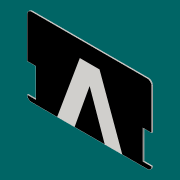
# Autodesk Inventor part: card-00
Saved by Autodesk Inventor 2016 (Build 200138000, 138)
## iProperties
Created: 2015-10-05
Part Number: card-00
Material: ABS Plastic
Document SubType Name: Modeling
Designer: Sawaiz
Density: 1.06 g/cm^3
Appearance: Smooth - White
Mass: 3.5118 g
Surface Area: 89.4505 cm^2
Volume: 3.31302 cm^3
Author: Sawaiz
Autodesk Inventor part; units mm, degrees
ref_plane "YZ Plane" through (0, 0, 0) normal (1, 0, 0) x (0, 1, 0)
ref_plane "XZ Plane" through (0, 0, 0) normal (0, 1, 0) x (-1, 0, 0)
ref_plane "XY Plane" through (0, 0, 0) normal (0, 0, 1) x (1, 0, 0)
sketch "Sketch1" plane through (0, 0, 0) normal (0, 1, 0) x (-1, 0, 0)
  line L0 (42.8, -26.99) -> (-42.8, -26.99)
  line L1 (-42.8, -26.99) -> (-42.8, 26.99)
  line L2 (-42.8, 26.99) -> (42.8, 26.99)
  line L3 (42.8, 26.99) -> (42.8, -26.99)
  line L4 (42.8, -26.99) -> (-42.8, 26.99) construction
  line L5 (-42.8, -26.99) -> (42.8, 26.99) construction
  point P0 (0, 0)
  dimension "d0" = 85.6
  dimension "d1" = 53.98
  constraints: 12 end point, 2 midpoint, 2 parallel, 1 horizontal, 1 perpendicular
  measures "d0" distance of L1.end L2.end
  measures "d1" distance of L0.end L1.end
extrude "Extrusion1" add sketch "Sketch1" along normal blind 0.76
fillet "Fillet1" radius 2.88 4 edges at (42.8, 0.38, 26.99) (42.8, 0.38, -26.99) (-42.8, 0.38, 26.99) (-42.8, 0.38, -26.99)
sketch "Sketch2" plane through (0, 0, 0) normal (0, -1, 0) x (1, 0, 0)
  arc A0 (-42.8, -24.11) -> (-39.92, -26.99) centre (-39.92, -24.11) ccw projected
  line L0 (-39.92, -26.99) -> (39.92, -26.99) projected
  arc A1 (39.92, -26.99) -> (42.8, -24.11) centre (39.92, -24.11) ccw projected
  line L1 (42.8, -24.11) -> (42.8, 24.11) projected
  arc A2 (42.8, 24.11) -> (39.92, 26.99) centre (39.92, 24.11) ccw projected
  line L2 (39.92, 26.99) -> (-39.92, 26.99) projected
  arc A3 (-39.92, 26.99) -> (-42.8, 24.11) centre (-39.92, 24.11) ccw projected
  line L3 (-42.8, 24.11) -> (-42.8, -24.11) projected
  line L4 (-42.8, 24.11) -> (-42.8, -24.11) projected
  line L5 (-42.8, -3.99) -> (-37.212, -3.99)
  line L6 (-37.212, -3.99) -> (-37.212, -23.99)
  line L7 (-37.212, -23.99) -> (-42.8, -23.99)
  line L8 (-42.8, -23.99) -> (-42.8, -3.99)
  line L9 (42.8, 24.11) -> (42.8, -24.11) projected
  line L10 (42.8, -23.99) -> (37.212, -23.99)
  line L11 (37.212, -23.99) -> (37.212, -3.99)
  line L12 (37.212, -3.99) -> (42.8, -3.99)
  line L13 (42.8, -3.99) -> (42.8, -23.99)
  point P0 (0, 0)
  dimension "d5" = 5.588
  dimension "d6" = 5.588
  dimension "d7" = 3
  dimension "d8" = 3
  dimension "d9" = 20
  dimension "d10" = 20
  constraints: 16 end point, 4 parallel, 2 horizontal, 2 perpendicular, 2 point on line
  measures "d5" distance between parallel lines of L6 L3
  measures "d6" distance of L11.end L12.end
  measures "d7" distance between parallel lines of L0 L7
  measures "d8" distance between parallel lines of L0 L10
  measures "d9" distance between parallel lines of L10 L12
  measures "d10" distance between parallel lines of L7 L5
extrude "Extrusion2" cut sketch "Sketch2" against normal through all contours L3 L5 L6 L7 | L10 L11 L12 L1
sketch "Sketch3" plane through (42.8, 0, 24.11) normal (1, 0, 0) x (0, 0, -1)
  line L0 (51.1, 0) -> (51.1, 0.76) projected
  line L1 (51.1, 0) -> (51.1, 0.76)
  line L2 (48.1, 0.76) -> (48.1, 0)
  line L3 (48.1, 0) -> (51.1, 0.76) construction
  line L4 (51.1, 0) -> (48.1, 0.76) construction
  line L5 (51.1, 0) -> (48.22, 0) projected
  arc A0 (48.1489, 0.76) -> (48.1489, 0) centre (49.6, 0.38) ccw
  arc A1 (51.0511, 0) -> (51.0511, 0.76) centre (49.6, 0.38) ccw
  line L6 (48.1, 0) -> (48.1489, 0)
  line L7 (51.0511, 0) -> (51.1, 0)
  line L8 (51.1, 0.76) -> (51.0511, 0.76)
  line L9 (48.1489, 0.76) -> (48.1, 0.76)
  point P0 (24.11, 0)
  point P1 (48.1, 0.38)
  point P2 (51.1, 0.38)
  dimension "d14" = 3
  dimension "d15" = 0.76
  dimension "d16" = 1.5
  dimension "d17" = 1.5
  dimension "d18" = 1.5
  constraints: 16 end point, 6 point on circle, 5 parallel, 4 midpoint, 3 collinear, 2 centre point, 2 horizontal, 2 perpendicular, 1 point on line
  measures "d14" distance of L2.start L1.end
  measures "d15" distance of L0.start L1.end
  measures "d16" radius of A0
  measures "d17" distance from line of L0 A0.centre
  measures "d18" radius of A1
extrude "Extrusion3" cut sketch "Sketch3" against normal up to surface (5.588 mm away)
mirror "Mirror1" about plane through (0, 0, 0) normal (1, 0, 0) of "Extrusion3"
sketch "Sketch4" plane through (0, 0, 0) normal (0, -1, 0) x (1, 0, 0)
  line L0 (-37.212, -24.0389) -> (-42.8, -24.0389) projected
  line L1 (-42.8, -24.0389) -> (-42.8, -24.11) projected
  arc A0 (-42.8, -24.11) -> (-40.4486, -26.9411) centre (-39.92, -24.11) ccw projected
  line L2 (-40.4486, -26.9411) -> (-37.212, -26.9411) projected
  line L3 (-37.212, -26.9411) -> (-37.212, -26.99) projected
  line L4 (-37.212, -26.99) -> (37.212, -26.99) projected
  line L5 (37.212, -26.99) -> (37.212, -26.9411) projected
  line L6 (37.212, -26.9411) -> (40.4486, -26.9411) projected
  arc A1 (40.4486, -26.9411) -> (42.8, -24.11) centre (39.92, -24.11) ccw projected
  line L7 (42.8, -24.11) -> (42.8, -24.0389) projected
  line L8 (42.8, -24.0389) -> (37.212, -24.0389) projected
  line L9 (37.212, -24.0389) -> (37.212, -3.99) projected
  line L10 (37.212, -3.99) -> (42.8, -3.99) projected
  line L11 (42.8, -3.99) -> (42.8, 24.11) projected
  arc A2 (42.8, 24.11) -> (39.92, 26.99) centre (39.92, 24.11) ccw projected
  line L12 (39.92, 26.99) -> (-39.92, 26.99) projected
  arc A3 (-39.92, 26.99) -> (-42.8, 24.11) centre (-39.92, 24.11) ccw projected
  line L13 (-42.8, 24.11) -> (-42.8, -3.99) projected
  line L14 (-42.8, -3.99) -> (-37.212, -3.99) projected
  line L15 (-37.212, -3.99) -> (-37.212, -24.0389) projected
  line L16 (39.92, 26.99) -> (-39.92, 26.99) projected
  line L17 (42.8, -3.99) -> (42.8, 24.11) projected
  line L18 (-42.8, 24.11) -> (-42.8, -3.99) projected
  line L19 (-42.8, 26.99) -> (42.8, 26.99) construction
  line L20 (42.8, 26.99) -> (42.8, -27.0263) construction
  line L21 (42.8, -27.0263) -> (-42.8, -27.0263) construction
  line L22 (-42.8, -27.0263) -> (-42.8, 26.99) construction
  point P0 (0, 0)
  constraints: 3 collinear, 2 other
decal "Decal1"
sketch "Sketch5" plane through (0, 0.76, 0) normal (0, 1, 0) x (1, 0, 0)
  line L0 (-42.8, 24.0389) -> (-37.212, 24.0389) projected
  line L1 (-37.212, 24.0389) -> (-37.212, 3.99) projected
  line L2 (-37.212, 3.99) -> (-42.8, 3.99) projected
  line L3 (-42.8, 3.99) -> (-42.8, -24.11) projected
  arc A0 (-42.8, -24.11) -> (-39.92, -26.99) centre (-39.92, -24.11) ccw projected
  line L4 (-39.92, -26.99) -> (39.92, -26.99) projected
  arc A1 (39.92, -26.99) -> (42.8, -24.11) centre (39.92, -24.11) ccw projected
  line L5 (42.8, -24.11) -> (42.8, 3.99) projected
  line L6 (42.8, 3.99) -> (37.212, 3.99) projected
  line L7 (37.212, 3.99) -> (37.212, 24.0389) projected
  line L8 (37.212, 24.0389) -> (42.8, 24.0389) projected
  line L9 (42.8, 24.0389) -> (42.8, 24.11) projected
  arc A2 (42.8, 24.11) -> (40.4486, 26.9411) centre (39.92, 24.11) ccw projected
  line L10 (40.4486, 26.9411) -> (37.212, 26.9411) projected
  line L11 (37.212, 26.9411) -> (37.212, 26.99) projected
  line L12 (37.212, 26.99) -> (-37.212, 26.99) projected
  line L13 (-37.212, 26.99) -> (-37.212, 26.9411) projected
  line L14 (-37.212, 26.9411) -> (-40.4486, 26.9411) projected
  arc A3 (-40.4486, 26.9411) -> (-42.8, 24.11) centre (-39.92, 24.11) ccw projected
  line L15 (-42.8, 24.11) -> (-42.8, 24.0389) projected
  line L16 (-42.8, 3.99) -> (-42.8, -24.11) projected
  line L17 (-42.8, 27.0263) -> (42.8, 27.0263) construction
  line L18 (42.8, 27.0263) -> (42.8, -26.99) construction
  line L19 (42.8, -26.99) -> (-42.8, -26.99) construction
  line L20 (-42.8, -26.99) -> (-42.8, 27.0263) construction
  point P0 (0, 0)
  constraints: 3 collinear, 2 other
decal "Decal2"
equation "\"d0\" = cardWidth"
equation "\"d1\" = cardHeight"
equation "\"d2\" = cardThickness"
equation "\"d4\" = cardFillet"
equation "\"d5\" = spoolThickness"
equation "\"d6\" = spoolThickness"
equation "\"d7\" = cardPinDiameter"
equation "\"d8\" = cardPinDiameter"
equation "\"d9\" = cardCutoutHeight"
equation "\"d10\" = cardCutoutHeight"
equation "\"d11\" = cardThickness"
equation "\"d14\" = cardPinDiameter"
equation "\"d15\" = cardThickness"
equation "\"d16\" = 0.5 * cardPinDiameter"
equation "\"d18\" = 0.5 * cardPinDiameter"
equation "\"d19\" = cardThickness"
equation "\"materialThickness\" = 3.175"
equation "\"laserKerf\" = 0.1"
equation "\"spoolDiameter\" = 95"
equation "\"cardPinDiameter\" = 3"
equation "\"centeralShaftDiameter\" = 8"
equation "\"cardWidth\" = 85.6"
equation "\"cardHeight\" = 53.98"
equation "\"cardThickness\" = 0.76"
equation "\"cardFillet\" = 2.88"
equation "\"cardCutoutHeight\" = 20"
equation "\"d13\" = cardPinDiameter"
equation "\"cardClearence\" = 0.5"
equation "\"bearingWidth\" = 8"
equation "\"bearingOd\" = 22"
equation "\"axleHeight\" = 95"
equation "\"nutTrapDepth\" = 2.5"
equation "\"nutTrapwidth\" = 5.5"
equation "\"nutTrapClearence\" = 2"
equation "\"magnetLength\" = 3"
equation "\"magnetDiameter\" = 6"
equation "\"magnetProtusion\" = 0.25"
equation "\"spoolThickness\" = 5.588"
body "Solid1"
